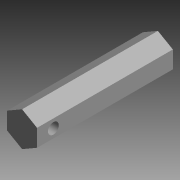
# Autodesk Inventor part: tensioners
Saved by Autodesk Inventor 2015 (Build 190159000, 159)
## iProperties
Created: 2014-05-14
Part Number: tensioners
Material: Generic
Document SubType Name: Modeling
Designer: Jascha
Density: 1 g/cm^3
Appearance: Default
Author: Jascha
Autodesk Inventor part; units mm, degrees
ref_plane "YZ Plane" through (0, 0, 0) normal (1, 0, 0) x (0, 1, 0)
ref_plane "XZ Plane" through (0, 0, 0) normal (0, 1, 0) x (-1, 0, 0)
ref_plane "XY Plane" through (0, 0, 0) normal (0, 0, 1) x (1, 0, 0)
sketch "Sketch1" plane through (0, 0, 0) normal (0, 0, 1) x (1, 0, 0)
  line L0 (2.794, -1.6131) -> (0, -3.2262)
  line L1 (0, -3.2262) -> (-2.794, -1.6131)
  line L2 (-2.794, -1.6131) -> (-2.794, 1.6131)
  line L3 (-2.794, 1.6131) -> (0, 3.2262)
  line L4 (0, 3.2262) -> (2.794, 1.6131)
  line L5 (2.794, 1.6131) -> (2.794, -1.6131)
  point P0 (0, 0)
  point P1 (0, 0)
  point P2 (2.794, 0)
  dimension "d0" = 5.588
  constraints: 12 end point, 1 coincident, 1 horizontal alignment, 1 midpoint, 13 other
  measures "d0" distance between parallel lines of L5 L2
extrude "Extrusion1" add sketch "Sketch1" along normal mid plane 25.4
sketch "Sketch2" plane through (2.794, -1.6131, 12.7) normal (1, 0, 0) x (0, 0, -1)
  line L0 (0, 0) -> (0, 3.2262) construction
  circle A0 centre (3.0551, 1.6131) radius 1.016
  point P0 (12.7, 1.6131)
  dimension "d3" = 2.032
  dimension "d4" = 3.0551
  constraints: 1 centre point, 1 horizontal alignment
  measures "d3" diameter of A0
  measures "d4" distance from line of L0 A0.centre
extrude "Extrusion2" cut sketch "Sketch2" against normal through all
sketch "Sketch3" plane through (0, 0, -12.7) normal (0, 0, -1) x (-1, 0, 0)
  circle A0 centre (0, 0) radius 1.397
  dimension "d9" = 2.794
  constraints: 1 centre point, 1 coincident
  measures "d9" diameter of A0
extrude "Extrusion3" cut sketch "Sketch3" against normal blind 19.05
body "Solid1"
